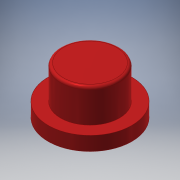
# Autodesk Inventor part: NØD-knap
Saved by Autodesk Inventor 2016 (Build 200138000, 138)
## iProperties
Created: 2016-03-15
Part Number: NØD-knap
Material: Generic
Document SubType Name: Modeling
Designer: Mathias L. Kjeldgaard
Density: 1 g/cm^3
Appearance: Light Red
Author: Mathias L. Kjeldgaard
Autodesk Inventor part; units mm, degrees
ref_plane "YZ Plane" through (0, 0, 0) normal (1, 0, 0) x (0, 1, 0)
ref_plane "XZ Plane" through (0, 0, 0) normal (0, 1, 0) x (-1, 0, 0)
ref_plane "XY Plane" through (0, 0, 0) normal (0, 0, 1) x (1, 0, 0)
sketch "Sketch1" plane through (0, 0, 0) normal (0, 0, 1) x (1, 0, 0)
  circle A0 centre (0, 0) radius 7.5
  circle A1 centre (0, 0) radius 1.6
  dimension "d0" = 15
  dimension "d1" = 3.2
  constraints: 2 centre point, 2 coincident
  measures "d0" diameter of A0
  measures "d1" diameter of A1
extrude "Ydre diameter" add sketch "Sketch1" along normal blind 4.5
sketch "Sketch2" plane through (0, 0, 4.5) normal (0, 0, 1) x (1, 0, 0)
  circle A0 centre (0, 0) radius 5.25
  dimension "d4" = 10.5
  constraints: 1 centre point, 1 coincident
  measures "d4" diameter of A0
extrude "Indre diameter" add sketch "Sketch2" along normal blind 6
fillet "Fillet1" radius 0.5 1 edges at (-5.25, 0, 10.5)
sketch "Sketch3" plane through (0, 0, 4.5) normal (0, 0, -1) x (-1, 0, 0)
  circle A0 centre (0, 0) radius 1.6 projected
extrude "Reducering af indre hul" add sketch "Sketch3" along normal blind 3.5
body "Solid1"
